Autodesk Inventor part; units mm, degrees
(part 2 of 2)
  spline S234 degree 2 poles (-105.034, 86.8201) (-105.034, 87.0103) (-105.0735, 87.1906) (-105.1353, 87.287) knots 0 0 0 1 2 2 2
  spline S235 degree 2 poles (-105.1353, 87.287) (-105.1945, 87.3808) (-105.3847, 87.4574) (-105.528, 87.4574) knots 0 0 0 1 2 2 2
  spline S236 degree 2 poles (-103.4655, 89.6705) (-103.4309, 89.6236) (-103.3074, 89.4655) (-103.2704, 89.3914) knots 0 0 0 1 2 2 2
  spline S237 degree 2 poles (-103.2704, 89.3914) (-103.2161, 89.2902) (-103.1592, 89.1) (-103.1592, 88.9271) knots 0 0 0 1 2 2 2
  spline S238 degree 2 poles (-103.1592, 88.9271) (-103.1592, 88.7863) (-103.2655, 88.5319) (-103.3618, 88.4355) knots 0 0 0 1 2 2 2
  spline S239 degree 2 poles (-103.3618, 88.4355) (-103.4556, 88.3441) (-103.7323, 88.233) (-103.8854, 88.233) knots 0 0 0 1 2 2 2
  spline S240 degree 2 poles (-103.8854, 88.233) (-104.1225, 88.233) (-104.4585, 88.4331) (-104.5548, 88.6504) knots 0 0 0 1 2 2 2
  spline S241 degree 2 poles (-104.5548, 88.6504) (-104.6437, 88.8431) (-104.7104, 89.3667) (-104.7277, 89.6705) knots 0 0 0 1 2 2 2
  line L249 (-104.7277, 89.6705) -> (-104.8018, 89.6705)
  spline S242 degree 2 poles (-104.8018, 89.6705) (-104.9352, 89.6705) (-105.1007, 89.589) (-105.1476, 89.5149) knots 0 0 0 1 2 2 2
  spline S243 degree 2 poles (-105.1476, 89.5149) (-105.1945, 89.4408) (-105.2242, 89.2284) (-105.2242, 89.1148) knots 0 0 0 1 2 2 2
  spline S244 degree 2 poles (-105.2242, 89.1148) (-105.2242, 88.9814) (-105.1451, 88.6208) (-105.0686, 88.4405) knots 0 0 0 1 2 2 2
  line L250 (-105.0686, 88.4405) -> (-105.0686, 88.4182)
  line L251 (-105.0686, 88.4182) -> (-105.4613, 88.4182)
  spline S245 degree 2 poles (-105.4613, 88.4182) (-105.4909, 88.5245) (-105.565, 88.9221) (-105.565, 89.1173) knots 0 0 0 1 2 2 2
  spline S246 degree 2 poles (-105.565, 89.1173) (-105.565, 89.3544) (-105.4909, 89.6779) (-105.3946, 89.8064) knots 0 0 0 1 2 2 2
  spline S247 degree 2 poles (-105.3946, 89.8064) (-105.3007, 89.9324) (-105.0019, 90.0559) (-104.787, 90.0559) knots 0 0 0 1 2 2 2
  line L252 (-104.787, 90.0559) -> (-103.2235, 90.0559)
  line L253 (-103.2235, 90.0559) -> (-103.2235, 89.6705)
  line L254 (-103.2235, 89.6705) -> (-103.4655, 89.6705)
  line L255 (-103.7866, 89.6705) -> (-104.4214, 89.6705)
  spline S248 degree 2 poles (-104.4214, 89.6705) (-104.4091, 89.5322) (-104.3671, 89.1148) (-104.3276, 88.9839) knots 0 0 0 1 2 2 2
  spline S249 degree 2 poles (-104.3276, 88.9839) (-104.2806, 88.8307) (-104.0855, 88.6307) (-103.9126, 88.6307) knots 0 0 0 1 2 2 2
  spline S250 degree 2 poles (-103.9126, 88.6307) (-103.715, 88.6307) (-103.5149, 88.853) (-103.5149, 89.0654) knots 0 0 0 1 2 2 2
  spline S251 degree 2 poles (-103.5149, 89.0654) (-103.5149, 89.2457) (-103.6705, 89.5421) (-103.7866, 89.6705) knots 0 0 0 1 2 2 2
  spline S252 degree 2 poles (-103.179, 91.2884) (-103.179, 90.9747) (-103.5372, 90.6215) (-103.9249, 90.6215) knots 0 0 0 1 2 2 2
  line L256 (-103.9249, 90.6215) -> (-105.1921, 90.6215)
  line L257 (-105.1921, 90.6215) -> (-105.1921, 90.3621)
  line L258 (-105.1921, 90.3621) -> (-105.5107, 90.3621)
  line L259 (-105.5107, 90.3621) -> (-105.5107, 90.6215)
  line L260 (-105.5107, 90.6215) -> (-106.1677, 90.6215)
  line L261 (-106.1677, 90.6215) -> (-106.1677, 91.0068)
  line L262 (-106.1677, 91.0068) -> (-105.5107, 91.0068)
  line L263 (-105.5107, 91.0068) -> (-105.5107, 91.7157)
  line L264 (-105.5107, 91.7157) -> (-105.1921, 91.7157)
  line L265 (-105.1921, 91.7157) -> (-105.1921, 91.0068)
  line L266 (-105.1921, 91.0068) -> (-104.1028, 91.0068)
  spline S253 degree 2 poles (-104.1028, 91.0068) (-103.9299, 91.0068) (-103.7397, 91.0192) (-103.6582, 91.0612) knots 0 0 0 1 2 2 2
  spline S254 degree 2 poles (-103.6582, 91.0612) (-103.5866, 91.0957) (-103.5149, 91.2513) (-103.5149, 91.3847) knots 0 0 0 1 2 2 2
  spline S255 degree 2 poles (-103.5149, 91.3847) (-103.5149, 91.4786) (-103.5717, 91.654) (-103.589, 91.6935) knots 0 0 0 1 2 2 2
  line L267 (-103.589, 91.6935) -> (-103.589, 91.7157)
  line L268 (-103.589, 91.7157) -> (-103.2432, 91.7157)
  spline S256 degree 2 poles (-103.2432, 91.7157) (-103.2136, 91.607) (-103.179, 91.3847) (-103.179, 91.2884) knots 0 0 0 1 2 2 2
  spline S257 degree 2 poles (-103.179, 92.6914) (-103.179, 92.3777) (-103.5372, 92.0245) (-103.9249, 92.0245) knots 0 0 0 1 2 2 2
  line L269 (-103.9249, 92.0245) -> (-105.1921, 92.0245)
  line L270 (-105.1921, 92.0245) -> (-105.1921, 91.7651)
  line L271 (-105.1921, 91.7651) -> (-105.5107, 91.7651)
  line L272 (-105.5107, 91.7651) -> (-105.5107, 92.0245)
  line L273 (-105.5107, 92.0245) -> (-106.1677, 92.0245)
  line L274 (-106.1677, 92.0245) -> (-106.1677, 92.4098)
  line L275 (-106.1677, 92.4098) -> (-105.5107, 92.4098)
  line L276 (-105.5107, 92.4098) -> (-105.5107, 93.1187)
  line L277 (-105.5107, 93.1187) -> (-105.1921, 93.1187)
  line L278 (-105.1921, 93.1187) -> (-105.1921, 92.4098)
  line L279 (-105.1921, 92.4098) -> (-104.1028, 92.4098)
  spline S258 degree 2 poles (-104.1028, 92.4098) (-103.9299, 92.4098) (-103.7397, 92.4221) (-103.6582, 92.4641) knots 0 0 0 1 2 2 2
  spline S259 degree 2 poles (-103.6582, 92.4641) (-103.5866, 92.4987) (-103.5149, 92.6543) (-103.5149, 92.7877) knots 0 0 0 1 2 2 2
  spline S260 degree 2 poles (-103.5149, 92.7877) (-103.5149, 92.8816) (-103.5717, 93.0569) (-103.589, 93.0965) knots 0 0 0 1 2 2 2
  line L280 (-103.589, 93.0965) -> (-103.589, 93.1187)
  line L281 (-103.589, 93.1187) -> (-103.2432, 93.1187)
  spline S261 degree 2 poles (-103.2432, 93.1187) (-103.2136, 93.01) (-103.179, 92.7877) (-103.179, 92.6914) knots 0 0 0 1 2 2 2
  spline S262 degree 2 poles (-103.1716, 94.3957) (-103.1716, 93.8473) (-103.7866, 93.2447) (-104.3547, 93.2447) knots 0 0 0 1 2 2 2
  spline S263 degree 2 poles (-104.3547, 93.2447) (-104.913, 93.2447) (-105.5749, 93.83) (-105.5749, 94.3018) knots 0 0 0 1 2 2 2
  spline S264 degree 2 poles (-105.5749, 94.3018) (-105.5749, 94.5142) (-105.4514, 94.8428) (-105.3205, 94.9638) knots 0 0 0 1 2 2 2
  spline S265 degree 2 poles (-105.3205, 94.9638) (-105.1896, 95.0873) (-104.8117, 95.2182) (-104.5375, 95.2182) knots 0 0 0 1 2 2 2
  line L282 (-104.5375, 95.2182) -> (-104.3276, 95.2182)
  line L283 (-104.3276, 95.2182) -> (-104.3276, 93.6349)
  spline S266 degree 2 poles (-104.3276, 93.6349) (-103.9299, 93.6349) (-103.5075, 94.0351) (-103.5075, 94.3907) knots 0 0 0 1 2 2 2
  spline S267 degree 2 poles (-103.5075, 94.3907) (-103.5075, 94.5167) (-103.5643, 94.7612) (-103.6088, 94.86) knots 0 0 0 1 2 2 2
  spline S268 degree 2 poles (-103.6088, 94.86) (-103.6582, 94.9638) (-103.7446, 95.107) (-103.7842, 95.154) knots 0 0 0 1 2 2 2
  line L284 (-103.7842, 95.154) -> (-103.7842, 95.1762)
  line L285 (-103.7842, 95.1762) -> (-103.3643, 95.1762)
  spline S269 degree 2 poles (-103.3643, 95.1762) (-103.3371, 95.1095) (-103.258, 94.907) (-103.2358, 94.8279) knots 0 0 0 1 2 2 2
  spline S270 degree 2 poles (-103.2358, 94.8279) (-103.2037, 94.7168) (-103.1716, 94.534) (-103.1716, 94.3957) knots 0 0 0 1 2 2 2
  spline S271 degree 2 poles (-104.6215, 94.8428) (-104.7771, 94.8378) (-105.0043, 94.7736) (-105.0809, 94.7118) knots 0 0 0 1 2 2 2
  spline S272 degree 2 poles (-105.0809, 94.7118) (-105.1674, 94.6452) (-105.2588, 94.4352) (-105.2588, 94.2796) knots 0 0 0 1 2 2 2
  spline S273 degree 2 poles (-105.2588, 94.2796) (-105.2588, 94.1264) (-105.1674, 93.9116) (-105.0784, 93.8226) knots 0 0 0 1 2 2 2
  spline S274 degree 2 poles (-105.0784, 93.8226) (-104.9871, 93.7362) (-104.7672, 93.6473) (-104.6215, 93.6349) knots 0 0 0 1 2 2 2
  line L286 (-104.6215, 93.6349) -> (-104.6215, 94.8428)
  line L287 (-105.0982, 96.8212) -> (-105.0982, 96.8015)
  spline S275 degree 2 poles (-105.0982, 96.8015) (-105.1106, 96.757) (-105.1155, 96.6607) (-105.1155, 96.594) knots 0 0 0 1 2 2 2
  spline S276 degree 2 poles (-105.1155, 96.594) (-105.1155, 96.4384) (-104.9796, 96.1321) (-104.8463, 95.9938) knots 0 0 0 1 2 2 2
  line L288 (-104.8463, 95.9938) -> (-103.2235, 95.9938)
  line L289 (-103.2235, 95.9938) -> (-103.2235, 95.6085)
  line L290 (-103.2235, 95.6085) -> (-105.5107, 95.6085)
  line L291 (-105.5107, 95.6085) -> (-105.5107, 95.9938)
  line L292 (-105.5107, 95.9938) -> (-105.1698, 95.9938)
  spline S277 degree 2 poles (-105.1698, 95.9938) (-105.3576, 96.2037) (-105.5107, 96.5174) (-105.5107, 96.6656) knots 0 0 0 1 2 2 2
  spline S278 degree 2 poles (-105.5107, 96.6656) (-105.5107, 96.7249) (-105.5058, 96.7842) (-105.4983, 96.8212) knots 0 0 0 1 2 2 2
  line L293 (-105.4983, 96.8212) -> (-105.0982, 96.8212)
  line L294 (-105.5107, 98.9158) -> (-102.3812, 97.6857)
  line L295 (-102.3812, 97.6857) -> (-102.3812, 97.2732)
  line L296 (-102.3812, 97.2732) -> (-103.3346, 97.6833)
  line L297 (-103.3346, 97.6833) -> (-105.5107, 96.8533)
  line L298 (-105.5107, 96.8533) -> (-105.5107, 97.2683)
  line L299 (-105.5107, 97.2683) -> (-103.8163, 97.8932)
  line L300 (-103.8163, 97.8932) -> (-105.5107, 98.5157)
  line L301 (-105.5107, 98.5157) -> (-105.5107, 98.9158)
  spline S279 degree 2 poles (-90.7486, 89.4309) (-90.3312, 89.4309) (-89.6594, 89.0926) (-89.4716, 88.8085) knots 0 0 0 1 2 2 2
  spline S280 degree 2 poles (-89.4716, 88.8085) (-89.3259, 88.5763) (-89.2271, 88.0996) (-89.2271, 87.7291) knots 0 0 0 1 2 2 2
  line L302 (-89.2271, 87.7291) -> (-89.2271, 87.0276)
  line L303 (-89.2271, 87.0276) -> (-92.2751, 87.0276)
  line L304 (-92.2751, 87.0276) -> (-92.2751, 87.7217)
  spline S281 degree 2 poles (-92.2751, 87.7217) (-92.2751, 88.1515) (-92.1467, 88.6405) (-92.0331, 88.8134) knots 0 0 0 1 2 2 2
  spline S282 degree 2 poles (-92.0331, 88.8134) (-91.8379, 89.1074) (-91.1933, 89.4309) (-90.7486, 89.4309) knots 0 0 0 1 2 2 2
  spline S283 degree 2 poles (-90.7536, 89.0086) (-91.1043, 89.0086) (-91.6008, 88.7764) (-91.7416, 88.5467) knots 0 0 0 1 2 2 2
  spline S284 degree 2 poles (-91.7416, 88.5467) (-91.8379, 88.3837) (-91.9244, 88.0156) (-91.9244, 87.7415) knots 0 0 0 1 2 2 2
  line L305 (-91.9244, 87.7415) -> (-91.9244, 87.4327)
  line L306 (-91.9244, 87.4327) -> (-89.5779, 87.4327)
  line L307 (-89.5779, 87.4327) -> (-89.5779, 87.7415)
  spline S285 degree 2 poles (-89.5779, 87.7415) (-89.5779, 88.0107) (-89.6643, 88.4182) (-89.7804, 88.5837) knots 0 0 0 1 2 2 2
  spline S286 degree 2 poles (-89.7804, 88.5837) (-89.9237, 88.7961) (-90.3979, 89.0086) (-90.7536, 89.0086) knots 0 0 0 1 2 2 2
  spline S287 degree 2 poles (-89.1728, 91.0612) (-89.1728, 90.7648) (-89.3728, 90.2633) (-89.5729, 90.0806) knots 0 0 0 1 2 2 2
  spline S288 degree 2 poles (-89.5729, 90.0806) (-89.7705, 89.8978) (-90.3633, 89.6977) (-90.7486, 89.6977) knots 0 0 0 1 2 2 2
  spline S289 degree 2 poles (-90.7486, 89.6977) (-91.1315, 89.6977) (-91.6996, 89.8928) (-91.9096, 90.0781) knots 0 0 0 1 2 2 2
  spline S290 degree 2 poles (-91.9096, 90.0781) (-92.1146, 90.2609) (-92.3295, 90.7598) (-92.3295, 91.0686) knots 0 0 0 1 2 2 2
  spline S291 degree 2 poles (-92.3295, 91.0686) (-92.3295, 91.2217) (-92.285, 91.4909) (-92.2504, 91.6046) knots 0 0 0 1 2 2 2
  spline S292 degree 2 poles (-92.2504, 91.6046) (-92.2183, 91.7034) (-92.1269, 91.9084) (-92.0726, 92.0096) knots 0 0 0 1 2 2 2
  line L308 (-92.0726, 92.0096) -> (-91.5835, 92.0096)
  line L309 (-91.5835, 92.0096) -> (-91.5835, 91.9775)
  spline S293 degree 2 poles (-91.5835, 91.9775) (-91.6329, 91.9232) (-91.7712, 91.7552) (-91.8379, 91.6342) knots 0 0 0 1 2 2 2
  spline S294 degree 2 poles (-91.8379, 91.6342) (-91.9021, 91.5181) (-91.9837, 91.2439) (-91.9837, 91.0661) knots 0 0 0 1 2 2 2
  spline S295 degree 2 poles (-91.9837, 91.0661) (-91.9837, 90.871) (-91.8231, 90.5227) (-91.67, 90.3918) knots 0 0 0 1 2 2 2
  spline S296 degree 2 poles (-91.67, 90.3918) (-91.5144, 90.2633) (-91.0426, 90.1201) (-90.7486, 90.1201) knots 0 0 0 1 2 2 2
  spline S297 degree 2 poles (-90.7486, 90.1201) (-90.435, 90.1201) (-89.9829, 90.2707) (-89.8273, 90.4017) knots 0 0 0 1 2 2 2
  spline S298 degree 2 poles (-89.8273, 90.4017) (-89.6767, 90.5301) (-89.5235, 90.8734) (-89.5235, 91.0661) knots 0 0 0 1 2 2 2
  spline S299 degree 2 poles (-89.5235, 91.0661) (-89.5235, 91.2415) (-89.61, 91.5403) (-89.6742, 91.6564) knots 0 0 0 1 2 2 2
  spline S300 degree 2 poles (-89.6742, 91.6564) (-89.7384, 91.7676) (-89.8718, 91.9331) (-89.9187, 91.98) knots 0 0 0 1 2 2 2
  line L310 (-89.9187, 91.98) -> (-89.9187, 92.0096)
  line L311 (-89.9187, 92.0096) -> (-89.4346, 92.0096)
  spline S301 degree 2 poles (-89.4346, 92.0096) (-89.3877, 91.9084) (-89.3012, 91.7305) (-89.2617, 91.6046) knots 0 0 0 1 2 2 2
  spline S302 degree 2 poles (-89.2617, 91.6046) (-89.2172, 91.4712) (-89.1728, 91.2439) (-89.1728, 91.0612) knots 0 0 0 1 2 2 2
  line L312 (-89.2271, 94.7588) -> (-89.2271, 93.5781)
  line L313 (-89.2271, 93.5781) -> (-89.5383, 93.5781)
  line L314 (-89.5383, 93.5781) -> (-89.5383, 93.9659)
  line L315 (-89.5383, 93.9659) -> (-91.9639, 93.9659)
  line L316 (-91.9639, 93.9659) -> (-91.9639, 93.5781)
  line L317 (-91.9639, 93.5781) -> (-92.2751, 93.5781)
  line L318 (-92.2751, 93.5781) -> (-92.2751, 94.7588)
  line L319 (-92.2751, 94.7588) -> (-91.9639, 94.7588)
  line L320 (-91.9639, 94.7588) -> (-91.9639, 94.371)
  line L321 (-91.9639, 94.371) -> (-89.5383, 94.371)
  line L322 (-89.5383, 94.371) -> (-89.5383, 94.7588)
  line L323 (-89.5383, 94.7588) -> (-89.2271, 94.7588)
  line L324 (-89.2271, 97.4412) -> (-89.2271, 96.9867)
  line L325 (-89.2271, 96.9867) -> (-91.8552, 95.6381)
  line L326 (-91.8552, 95.6381) -> (-89.2271, 95.6381)
  line L327 (-89.2271, 95.6381) -> (-89.2271, 95.2602)
  line L328 (-89.2271, 95.2602) -> (-92.2751, 95.2602)
  line L329 (-92.2751, 95.2602) -> (-92.2751, 95.8357)
  line L330 (-92.2751, 95.8357) -> (-89.8619, 97.0633)
  line L331 (-89.8619, 97.0633) -> (-92.2751, 97.0633)
  line L332 (-92.2751, 97.0633) -> (-92.2751, 97.4412)
  line L333 (-92.2751, 97.4412) -> (-89.2271, 97.4412)
  spline S303 degree 2 poles (-156.612, 77.286) (-156.3526, 77.286) (-155.8859, 77.1012) (-155.7238, 76.9359) knots 0 0 0 1 2 2 2
  spline S304 degree 2 poles (-155.7238, 76.9359) (-155.5196, 76.7284) (-155.3089, 76.1676) (-155.3089, 75.7398) knots 0 0 0 1 2 2 2
  line L334 (-155.3089, 75.7398) -> (-155.3089, 75.2892)
  line L335 (-155.3089, 75.2892) -> (-153.8178, 75.2892)
  line L336 (-153.8178, 75.2892) -> (-153.8178, 74.7576)
  line L337 (-153.8178, 74.7576) -> (-157.8178, 74.7576)
  line L338 (-157.8178, 74.7576) -> (-157.8178, 75.7625)
  spline S305 degree 2 poles (-157.8178, 75.7625) (-157.8178, 76.119) (-157.7011, 76.6182) (-157.5682, 76.8095) knots 0 0 0 1 2 2 2
  spline S306 degree 2 poles (-157.5682, 76.8095) (-157.4159, 77.0331) (-156.9458, 77.286) (-156.612, 77.286) knots 0 0 0 1 2 2 2
  spline S307 degree 2 poles (-156.5958, 76.7317) (-156.8032, 76.7317) (-157.1079, 76.589) (-157.2052, 76.4432) knots 0 0 0 1 2 2 2
  spline S308 degree 2 poles (-157.2052, 76.4432) (-157.2894, 76.3167) (-157.3575, 75.9796) (-157.3575, 75.73) knots 0 0 0 1 2 2 2
  line L339 (-157.3575, 75.73) -> (-157.3575, 75.2892)
  line L340 (-157.3575, 75.2892) -> (-155.7627, 75.2892)
  line L341 (-155.7627, 75.2892) -> (-155.7627, 75.6522)
  spline S309 degree 2 poles (-155.7627, 75.6522) (-155.7627, 75.9764) (-155.8664, 76.3751) (-156.0026, 76.5048) knots 0 0 0 1 2 2 2
  spline S310 degree 2 poles (-156.0026, 76.5048) (-156.1225, 76.6247) (-156.4045, 76.7317) (-156.5958, 76.7317) knots 0 0 0 1 2 2 2
  spline S311 degree 2 poles (-155.3186, 80.2195) (-154.5601, 80.2195) (-153.7335, 79.4902) (-153.7335, 78.8808) knots 0 0 0 1 2 2 2
  spline S312 degree 2 poles (-153.7335, 78.8808) (-153.7335, 78.2552) (-154.586, 77.5388) (-155.3186, 77.5388) knots 0 0 0 1 2 2 2
  spline S313 degree 2 poles (-155.3186, 77.5388) (-156.0706, 77.5388) (-156.9037, 78.2778) (-156.9037, 78.8808) knots 0 0 0 1 2 2 2
  spline S314 degree 2 poles (-156.9037, 78.8808) (-156.9037, 79.4902) (-156.0739, 80.2195) (-155.3186, 80.2195) knots 0 0 0 1 2 2 2
  spline S315 degree 2 poles (-155.3186, 79.6976) (-155.9021, 79.6976) (-156.4693, 79.273) (-156.4693, 78.8808) knots 0 0 0 1 2 2 2
  spline S316 degree 2 poles (-156.4693, 78.8808) (-156.4693, 78.4885) (-155.9021, 78.0607) (-155.3186, 78.0607) knots 0 0 0 1 2 2 2
  spline S317 degree 2 poles (-155.3186, 78.0607) (-154.7513, 78.0607) (-154.1679, 78.4885) (-154.1679, 78.8808) knots 0 0 0 1 2 2 2
  spline S318 degree 2 poles (-154.1679, 78.8808) (-154.1679, 79.2697) (-154.7416, 79.6976) (-155.3186, 79.6976) knots 0 0 0 1 2 2 2
  line L342 (-156.8194, 84.3751) -> (-153.8178, 83.6133)
  line L343 (-153.8178, 83.6133) -> (-153.8178, 83.1466)
  line L344 (-153.8178, 83.1466) -> (-156.1322, 82.414)
  line L345 (-156.1322, 82.414) -> (-153.8178, 81.6847)
  line L346 (-153.8178, 81.6847) -> (-153.8178, 81.2211)
  line L347 (-153.8178, 81.2211) -> (-156.8194, 80.4529)
  line L348 (-156.8194, 80.4529) -> (-156.8194, 80.978)
  line L349 (-156.8194, 80.978) -> (-154.4953, 81.5096)
  line L350 (-154.4953, 81.5096) -> (-156.8194, 82.2195)
  line L351 (-156.8194, 82.2195) -> (-156.8194, 82.6377)
  line L352 (-156.8194, 82.6377) -> (-154.4953, 83.367)
  line L353 (-154.4953, 83.367) -> (-156.8194, 83.8662)
  line L354 (-156.8194, 83.8662) -> (-156.8194, 84.3751)
  spline S319 degree 2 poles (-153.7497, 86.1223) (-153.7497, 85.4026) (-154.5569, 84.6117) (-155.3024, 84.6117) knots 0 0 0 1 2 2 2
  spline S320 degree 2 poles (-155.3024, 84.6117) (-156.035, 84.6117) (-156.9037, 85.38) (-156.9037, 85.9991) knots 0 0 0 1 2 2 2
  spline S321 degree 2 poles (-156.9037, 85.9991) (-156.9037, 86.2778) (-156.7416, 86.709) (-156.5698, 86.8678) knots 0 0 0 1 2 2 2
  spline S322 degree 2 poles (-156.5698, 86.8678) (-156.398, 87.0299) (-155.9021, 87.2017) (-155.5423, 87.2017) knots 0 0 0 1 2 2 2
  line L355 (-155.5423, 87.2017) -> (-155.2667, 87.2017)
  line L356 (-155.2667, 87.2017) -> (-155.2667, 85.1239)
  spline S323 degree 2 poles (-155.2667, 85.1239) (-154.7449, 85.1239) (-154.1906, 85.649) (-154.1906, 86.1158) knots 0 0 0 1 2 2 2
  spline S324 degree 2 poles (-154.1906, 86.1158) (-154.1906, 86.2811) (-154.2651, 86.602) (-154.3235, 86.7317) knots 0 0 0 1 2 2 2
  spline S325 degree 2 poles (-154.3235, 86.7317) (-154.3883, 86.8678) (-154.5018, 87.0558) (-154.5536, 87.1174) knots 0 0 0 1 2 2 2
  line L357 (-154.5536, 87.1174) -> (-154.5536, 87.1466)
  line L358 (-154.5536, 87.1466) -> (-154.0026, 87.1466)
  spline S326 degree 2 poles (-154.0026, 87.1466) (-153.9669, 87.059) (-153.8632, 86.7932) (-153.834, 86.6895) knots 0 0 0 1 2 2 2
  spline S327 degree 2 poles (-153.834, 86.6895) (-153.7919, 86.5437) (-153.7497, 86.3038) (-153.7497, 86.1223) knots 0 0 0 1 2 2 2
  spline S328 degree 2 poles (-155.6525, 86.709) (-155.8567, 86.7025) (-156.1549, 86.6182) (-156.2554, 86.5372) knots 0 0 0 1 2 2 2
  spline S329 degree 2 poles (-156.2554, 86.5372) (-156.3689, 86.4496) (-156.4888, 86.1741) (-156.4888, 85.9699) knots 0 0 0 1 2 2 2
  spline S330 degree 2 poles (-156.4888, 85.9699) (-156.4888, 85.7689) (-156.3689, 85.4869) (-156.2522, 85.3702) knots 0 0 0 1 2 2 2
  spline S331 degree 2 poles (-156.2522, 85.3702) (-156.1322, 85.2568) (-155.8437, 85.1401) (-155.6525, 85.1239) knots 0 0 0 1 2 2 2
  line L359 (-155.6525, 85.1239) -> (-155.6525, 86.709)
  line L360 (-156.2781, 89.3054) -> (-156.2781, 89.2795)
  spline S332 degree 2 poles (-156.2781, 89.2795) (-156.2943, 89.2211) (-156.3008, 89.0947) (-156.3008, 89.0072) knots 0 0 0 1 2 2 2
  spline S333 degree 2 poles (-156.3008, 89.0072) (-156.3008, 88.803) (-156.1225, 88.401) (-155.9475, 88.2195) knots 0 0 0 1 2 2 2
  line L361 (-155.9475, 88.2195) -> (-153.8178, 88.2195)
  line L362 (-153.8178, 88.2195) -> (-153.8178, 87.7138)
  line L363 (-153.8178, 87.7138) -> (-156.8194, 87.7138)
  line L364 (-156.8194, 87.7138) -> (-156.8194, 88.2195)
  line L365 (-156.8194, 88.2195) -> (-156.3721, 88.2195)
  spline S334 degree 2 poles (-156.3721, 88.2195) (-156.6184, 88.495) (-156.8194, 88.9067) (-156.8194, 89.1012) knots 0 0 0 1 2 2 2
  spline S335 degree 2 poles (-156.8194, 89.1012) (-156.8194, 89.179) (-156.8129, 89.2568) (-156.8032, 89.3054) knots 0 0 0 1 2 2 2
  line L366 (-156.8032, 89.3054) -> (-156.2781, 89.3054)
  point P0 (0, 0)
  constraints: 16 other
extrude "Extrusion3" cut sketch "Sketch2" against normal blind 1.5 contours L15 L14 L13 L12 | L19 L18 L17 L16
extrude "Extrusion4" cut sketch "Sketch3" against normal blind 1.5
sketch "Sketch4" plane through (0, 2.5, 0) normal (0, 1, 0) x (1, 0, 0)
  line L0 (-85.1907, 14) -> (-155.1907, 14) projected
  line L1 (-129.1907, 14) -> (-111.1907, 14)
  line L2 (-111.1907, 14) -> (-111.1907, 17.5)
  line L3 (-111.1907, 17.5) -> (-129.1907, 17.5)
  line L4 (-129.1907, 17.5) -> (-129.1907, 14)
  line L5 (-155.1907, 14) -> (-155.1907, 34) projected
  line L6 (-85.1907, 40.3041) -> (-126.1907, 40.3041) projected
  line L7 (-105.6907, 40.3041) -> (-86.6907, 40.3041)
  line L8 (-86.6907, 40.3041) -> (-86.6907, 43.8041)
  line L9 (-86.6907, 43.8041) -> (-105.6907, 43.8041)
  line L10 (-105.6907, 43.8041) -> (-105.6907, 40.3041)
  point P0 (0, 0)
  point P1 (-129.1907, 15.75)
  point P2 (-86.6907, 40.3041)
  dimension "d88" = 18
  dimension "d89" = 3.5
  dimension "d90" = 26
  dimension "d91" = 19
  dimension "d92" = 3.5
  constraints: 16 end point, 4 parallel, 3 midpoint, 2 horizontal, 2 perpendicular, 1 point on line
  measures "d88" distance of L3.end L2.end
  measures "d89" distance of L2.end L1.end
  measures "d90" distance from line of L5 point (-129.191, 15.75)
  measures "d91" distance of L9.end L8.end
  measures "d92" distance of L8.end L7.end
extrude "Extrusion5" cut sketch "Sketch4" against normal through all
chamfer "Chamfer1" distance 8.5 angle 45 2 edges at (0, 2, 0) (-161.5, 2, 0)
sketch "Sketch5" plane through (0, 4, 0) normal (0, 1, 0) x (1, 0, 0)
  point P0 (0, 0)
sketch "Sketch8" plane through (0, 4, 0) normal (0, 1, 0) x (1, 0, 0)
  circle A0 centre (-80.75, 3) radius 1.25
  line L0 (-153, 0) -> (-8.5, 0) projected
  circle A1 centre (-6.3713, 6.3713) radius 1.25
  line L1 (0, 8.5) -> (-8.5, 0) projected
  circle A2 centre (-155.1287, 6.3713) radius 1.25
  line L2 (-153, 0) -> (-161.5, 8.5) projected
  circle A3 centre (-111.5, 102.5) radius 1.25
  circle A4 centre (-50, 102.5) radius 1.25
  line L3 (0, 105) -> (-161.5, 105) projected
  line L4 (-161.5, 105) -> (-161.5, 8.5) projected
  line L5 (0, 8.5) -> (0, 105) projected
  line L6 (-4.25, 4.25) -> (-6.3713, 6.3713) construction
  line L7 (-161.5, 105) -> (-161.5, 8.5) construction
  line L8 (-161.5, 8.5) -> (-153, 0) construction
  line L9 (-157.25, 4.25) -> (-155.1287, 6.3713) construction
  line L10 (-84, 100) -> (-12, 100) construction
  point P0 (0, 0)
  point P1 (-161.5, 40.7559)
  point P2 (-161.5, 35.7559)
  point P3 (-161.5, 22.128)
  dimension "d119" = 2.5
  dimension "d120" = 3
  dimension "d121" = 2.5
  dimension "d123" = 2.5
  dimension "d127" = 50
  dimension "d135" = 50
  dimension "d140" = 3
  dimension "d141" = 12.0208
  dimension "d142" = 6.0104
  dimension "d143" = 161.5
  dimension "d144" = 80.75
  dimension "d145" = 3
  dimension "d146" = 12.0208
  dimension "d147" = 6.0104
  dimension "d148" = 5
  dimension "d149" = 2.5
  dimension "d150" = 2.5
  dimension "d151" = 2.5
  constraints: 5 centre point, 4 coincident, 4 end point, 2 midpoint, 1 horizontal alignment, 1 point on line
  measures "d119" diameter of A0
  measures "d120" distance from line of L0 A0.centre
  measures "d121" diameter of A1
  measures "d123" diameter of A2
  measures "d127" distance from line of A3.centre L4
  measures "d135" distance from line of L5 A4.centre
  measures "d140" distance of L6.start L6.end
  measures "d141" distance of L1.start L0.end
  measures "d142" distance from line of L0.end L6
  measures "d143" distance from line of L5 point (-161.5, 22.128)
  measures "d144" distance from line of L7 A0.centre
  measures "d145" distance of L9.start L9.end
  measures "d146" distance of L0.start L2.end
  measures "d147" distance from line of L9 L2.end
  measures "d148" distance between parallel lines of L3 L10
  measures "d149" distance from line of L3 A4.centre
  measures "d150" diameter of A4
  measures "d151" diameter of A3
extrude "Extrusion8" cut sketch "Sketch8" against normal blind 10 contours A0 | A1 | A2 | A3 | A4
sketch "Sketch10" plane through (0, 4, 0) normal (0, 1, 0) x (1, 0, 0)
  circle A0 centre (-76, 45) radius 2.5
  line L0 (-70, 43) -> (-70, 87) projected
  line L1 (-26, 43) -> (-70, 43) projected
  circle A1 centre (-20, 45) radius 2.5
  circle A2 centre (-76, 85) radius 2.5
  circle A3 centre (-20, 85) radius 2.5
  line L2 (-70, 87) -> (-26, 87) construction
  line L3 (-70, 43) -> (-26, 87) construction
  line L4 (-26, 87) -> (-26, 43) construction
  line L5 (-70, 87) -> (-26, 43) construction
  point P0 (0, 0)
  point P1 (-48, 65)
  point P2 (-48, 65)
  dimension "d162" = 5
  dimension "d165" = 56
  dimension "d168" = 40
  dimension "d171" = 20
  dimension "d172" = 28
  constraints: 4 centre point, 4 end point, 2 midpoint, 1 horizontal, 1 vertical, 6 other
  measures "d162" diameter of A0
  measures "d165" distance of A0.centre A1.centre
  measures "d168" distance of A0.centre A2.centre
  measures "d171" vertical distance of A0.centre point (-48, 65)
  measures "d172" horizontal distance of A0.centre point (-48, 65)
extrude "Extrusion10" cut sketch "Sketch10" against normal blind 4
sketch "Sketch11" plane through (0, 0, 0) normal (0, -1, 0) x (1, 0, 0)
  line L0 (-131.6423, -82.601) -> (-148.6423, -82.601) projected
  line L1 (-148.6423, -82.601) -> (-148.6423, -50.601) projected
  line L2 (-131.6423, -50.601) -> (-131.6423, -82.601) projected
  line L3 (-148.6423, -50.601) -> (-131.6423, -50.601) projected
  line L4 (-154.2734, -93.5745) -> (-154.2734, -37.6262) construction
  line L5 (-154.2734, -37.6262) -> (-125.8797, -37.6262) construction
  line L6 (-125.8797, -37.6262) -> (-125.8797, -93.5745) construction
  line L7 (-125.8797, -93.5745) -> (-154.2734, -93.5745) construction
  line L8 (-192.1198, -160.8574) -> (-169.1198, -160.8574)
  line L9 (-148.6423, -55.0548) -> (-152.1207, -55.0548)
  line L10 (-152.1207, -55.0548) -> (-152.1207, -86.012)
  line L11 (-152.1207, -86.012) -> (-148.6423, -86.012)
  line L12 (-148.6423, -86.012) -> (-148.6423, -55.0548)
  line L13 (-131.6423, -86.012) -> (-128.3297, -86.012)
  line L14 (-128.3297, -86.012) -> (-128.3297, -44.7283)
  line L15 (-128.3297, -44.7283) -> (-131.6423, -44.7283)
  line L16 (-131.6423, -44.7283) -> (-131.6423, -86.012)
  line L17 (-152.1207, -50.3589) -> (-147.4248, -50.3589)
  line L18 (-147.4248, -50.3589) -> (-147.4248, -44.6615)
  line L19 (-147.4248, -44.6615) -> (-152.1207, -44.6615)
  line L20 (-152.1207, -44.6615) -> (-152.1207, -50.3589)
  circle A0 centre (-20, -45) radius 2.5 projected
  circle A1 centre (-76, -45) radius 2.5 projected
  circle A2 centre (-20, -85) radius 2.5 projected
  circle A3 centre (-76, -85) radius 2.5 projected
  circle A4 centre (-155.1287, -6.3713) radius 1.25 projected
  circle A5 centre (-111.5, -102.5) radius 1.25 projected
  circle A6 centre (-80.75, -3) radius 1.25 projected
  circle A7 centre (-50, -102.5) radius 1.25 projected
  circle A8 centre (-6.3713, -6.3713) radius 1.25 projected
  line L21 (-161.5, -8.5) -> (-153, 0) projected
  line L22 (-161.5, -105) -> (-161.5, -8.5) projected
  line L23 (0, -105) -> (-161.5, -105) projected
  line L24 (0, -8.5) -> (0, -105) projected
  line L25 (-8.5, 0) -> (0, -8.5) projected
  line L26 (-153, 0) -> (-8.5, 0) projected
  line L27 (-129.1907, -14) -> (-111.1907, -14) projected
  line L28 (-111.1907, -14) -> (-111.1907, -17.5) projected
  line L29 (-111.1907, -17.5) -> (-129.1907, -17.5) projected
  line L30 (-129.1907, -17.5) -> (-129.1907, -14) projected
  line L31 (-105.6907, -40.3041) -> (-86.6907, -40.3041) projected
  line L32 (-86.6907, -40.3041) -> (-86.6907, -43.8041) projected
  line L33 (-86.6907, -43.8041) -> (-105.6907, -43.8041) projected
  line L34 (-105.6907, -43.8041) -> (-105.6907, -40.3041) projected
  circle A9 centre (-68, -11) radius 2.5 projected
  line L35 (-131.6423, -82.601) -> (-148.6423, -82.601) projected
  line L36 (-148.6423, -82.601) -> (-148.6423, -50.601) projected
  line L37 (-148.6423, -50.601) -> (-131.6423, -50.601) projected
  line L38 (-131.6423, -50.601) -> (-131.6423, -82.601) projected
  circle A10 centre (-97.5813, -93) radius 3 projected
  circle A11 centre (-155.1907, -93) radius 2.5 projected
  circle A12 centre (-28, -11) radius 2.5 projected
  circle A13 centre (-119.8496, -94.6341) radius 5.5 projected
  line L39 (-26, -87) -> (-70, -87) projected
  line L40 (-70, -87) -> (-70, -43) projected
  line L41 (-70, -43) -> (-26, -43) projected
  line L42 (-26, -43) -> (-26, -87) projected
  line L43 (-133.76, -41.2853) -> (-146.8016, -41.2853)
  line L44 (-146.8016, -41.2853) -> (-146.8016, -47.5)
  line L45 (-146.8016, -47.5) -> (-133.76, -47.5)
  line L46 (-133.76, -47.5) -> (-133.76, -41.2853)
  circle A14 centre (-149.3294, -88.4843) radius 0.9
  circle A15 centre (-131.2884, -88.4843) radius 0.9
  circle A16 centre (-149.3294, -42.7693) radius 0.9
  circle A17 centre (-131.2884, -42.7693) radius 0.9
  line L47 (-148.6423, -82.601) -> (-131.6423, -82.601)
  line L48 (-131.6423, -82.601) -> (-131.6423, -87)
  line L49 (-131.6423, -87) -> (-148.6423, -87)
  line L50 (-148.6423, -87) -> (-148.6423, -82.601)
  line L51 (-145.8264, -87) -> (-134.2429, -87)
  line L52 (-134.2429, -87) -> (-134.2429, -88.4843)
  line L53 (-134.2429, -88.4843) -> (-145.8264, -88.4843)
  line L54 (-145.8264, -88.4843) -> (-145.8264, -87)
  circle A18 centre (-137.1913, -35.4246) radius 0.9
  circle A19 centre (-137.1913, -22.7246) radius 0.9
  circle A20 centre (-116.8713, -35.4246) radius 0.9
  circle A21 centre (-116.8713, -22.7246) radius 0.9
  point P0 (0, 0)
  dimension "d187" = 23
  dimension "d200" = 1.8
  dimension "d201" = 1.8
  dimension "d202" = 1.8
  dimension "d203" = 1.8
  dimension "d209" = 1.8
  dimension "d212" = 12.7
  dimension "d215" = 20.32
  constraints: 50 end point, 12 parallel, 8 centre point, 8 horizontal, 6 perpendicular, 3 point on line, 2 horizontal alignment, 2 vertical alignment, 1 vertical, 8 other
  measures "d187" distance of L8.start L8.end
  measures "d200" diameter of A14
  measures "d201" diameter of A15
  measures "d202" diameter of A16
  measures "d203" diameter of A17
  measures "d209" diameter of A18
  measures "d212" distance of A18.centre A19.centre
  measures "d215" distance of A18.centre A20.centre
extrude "Extrusion11" cut sketch "Sketch11" against normal blind 2.5 contours L16 L48 L49 L50 L12 L0 | L2 L16 L15 L14 L13 | L12 L11 L10 L9 L1 | L52 L53 L54 L49 | L20 L19 L18 L17 | L46 L45 L44 L43 | A14 | A15 | A16 | A17 | A18 | A20
sketch "Sketch12" plane through (0, 2.5, 0) normal (0, -1, 0) x (1, 0, 0)
  line L0 (-148.6423, -55.0548) -> (-148.6423, -82.601) projected
  line L1 (-148.6423, -82.601) -> (-131.6423, -82.601) projected
  line L2 (-131.6423, -82.601) -> (-131.6423, -50.601) projected
  line L3 (-149.0923, -55.0548) -> (-149.0923, -83.051)
  line L4 (-149.0923, -83.051) -> (-131.1923, -83.051)
  line L5 (-131.1923, -83.051) -> (-131.1923, -50.601)
  line L6 (-152.1207, -55.0548) -> (-148.6423, -55.0548) projected
  line L7 (-149.0923, -55.0548) -> (-148.6423, -55.0548)
  line L8 (-131.6423, -50.601) -> (-131.6423, -44.7283) projected
  line L9 (-131.6423, -50.601) -> (-131.1923, -50.601)
  point P0 (0, 0)
  dimension "d206" = 0.45
  constraints: 10 end point, 1 horizontal, 1 perpendicular, 2 other
  measures "d206" distance between parallel lines of L0 L3
extrude "Extrusion12" add sketch "Sketch12" along normal blind 2.5
body "Solid1"
